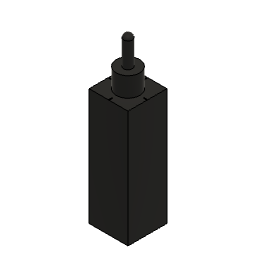
WW-PenMillReamerToolHolder (Autodesk Fusion 360 design; units mm, degrees)
Autodesk Fusion 360 part; units mm, degrees
sketch "Sketch1" plane through (0, 0, 0) normal (0, 1, 0) x (1, 0, 0) in component "Tool Holder - Whiteside"
  line L0 (0, 0) -> (25.4, 0)
  line L1 (25.4, 0) -> (25.4, -25.4)
  line L2 (25.4, -25.4) -> (0, -25.4)
  line L3 (0, -25.4) -> (0, 0)
  dimension "d1" = 25.4
  dimension "d2" = 25.4
  constraint horizontal L0
  constraint vertical L1
  constraint horizontal L2
  constraint vertical L3
  constraint coincident L0.start L3.end
  measures "d1" distance of L0.start L0.end
  measures "d2" distance of L0.start L2.end
extrude "Extrude1" add sketch "Sketch1" along normal blind 76.2 makes body 1 in component "Tool Holder - Whiteside"
sketch "Sketch2" plane through (0, 76.2, 0) normal (0, 1, 0) x (-1, 0, 0) in component "Tool Holder - Whiteside"
  line L0 (0, 25.4) -> (-25.4, 25.4)
  line L1 (-25.4, 25.4) -> (-25.4, 0)
  line L2 (-25.4, 0) -> (0, 0)
  line L3 (0, 0) -> (0, 25.4)
  line L4 (0, 25.4) -> (-12.7, 25.4)
  line L5 (-12.7, 25.4) -> (-12.7, 12.7)
  line L6 (-12.7, 12.7) -> (0, 12.7)
  line L7 (0, 12.7) -> (0, 25.4)
  circle A0 centre (-12.7, 12.7) radius 7.62
  dimension "d5" = 12.7
  dimension "d6" = 12.7
  dimension "d7" = 15.24
  constraint horizontal L4
  constraint vertical L5
  constraint horizontal L6
  constraint vertical L7
  constraint coincident L0.start L3.end
  constraint coincident L5.end L6.start
  measures "d5" distance of L0.start L4.end
  measures "d6" distance of L0.start L6.end
  measures "d7" diameter of A0
extrude "Extrude2" add sketch "Sketch2" along normal blind 12.7 contours L5 L6 A0 | L5 L6 A0 bodies 1 in component "Tool Holder - Whiteside"
sketch "Sketch3" plane through (0, 88.9, 0) normal (0, 1, 0) x (-1, 0, 0) in component "Tool Holder - Whiteside"
  circle A0 centre (-12.7, 12.7) radius 7.62
  circle A1 centre (-12.7, 12.7) radius 2.8575
  dimension "d10" = 5.715
  constraint concentric A0 A1
  measures "d10" diameter of A1
extrude "Extrude3" add sketch "Sketch3" along normal blind 19.05 contours A1 bodies 1 in component "Tool Holder - Whiteside"
chamfer "Chamfer1" distance 0.635 angle 45 1 edges at (15.3641, 107.95, 11.6667) on bodies 1 in component "Tool Holder - Whiteside"
chamfer "Chamfer2" distance 2.54 angle 45 3 edges at (25.4, 76.2, 12.7) (12.7, 76.2, 25.4) (0, 76.2, 12.7) on bodies 1 in component "Tool Holder - Whiteside"
fillet "Fillet1" radius 2.54 1 edges at (19.8043, 76.2, 15.4555) on bodies 1 in component "Tool Holder - Whiteside"
sketch "Sketch1 (2)" plane through (0, 0, 0) normal (0, 1, 0) x (1, 0, 0) in component "Milling Bit"
  circle A0 centre (-38.4906, 23.2969) radius 9.4361
  dimension "d17" = 18.8722
  measures "d17" diameter of A0
extrude "Extrude1'" add sketch "Sketch1 (2)" along normal blind 22.6568 separate body makes body 2 in component "Milling Bit"
sketch "Sketch2 (2)" plane through (0, 22.6568, 0) normal (0, 1, 0) x (-1, 0, 0) in component "Milling Bit"
  circle A0 centre (38.4906, -23.2969) radius 9.4361
  circle A1 centre (38.4906, -23.2969) radius 2.8702
  dimension "d20" = 5.7404
  constraint concentric A0 A1
  measures "d20" diameter of A1
extrude "Extrude2'" cut sketch "Sketch2 (2)" against normal blind 55.88 contours A1 bodies 2 in component "Milling Bit"
chamfer "Chamfer1'" distance 0.508 angle 45 1 edges at (-47.2881, 0, -19.8847) on bodies 2 in component "Milling Bit"
sketch "Sketch1 (3)" plane through (0, 111.5568, 0) normal (0, 1, 0) x (-1, 0, 0)
  circle A0 centre (-12.7067, 12.7059) radius 2.8702
  circle A1 centre (-12.7067, 12.7059) radius 9.4361
  line L0 (-12.7067, 12.7059) -> (-12.7067, 24.2231)
  line L1 (-12.7067, 24.2231) -> (-12.7067, 12.7059)
  line L2 (-12.7067, 1.8794) -> (-12.7067, 12.7059)
  line L3 (-12.7067, 12.7059) -> (-23.5469, 12.7059)
  line L4 (-12.7067, 12.7059) -> (-0.0671, 12.7059)
  line L5 (-12.7067, 12.7059) -> (-23.3575, 12.7059)
  line L6 (-23.3575, 12.7059) -> (-23.3575, 15.2459)
  line L7 (-23.3575, 15.2459) -> (-12.7067, 15.2459)
  line L8 (-12.7067, 15.2459) -> (-12.7067, 12.7059)
  line L9 (-12.7067, 12.7059) -> (-10.1667, 12.7059)
  line L10 (-10.1667, 12.7059) -> (-10.1667, 23.655)
  line L11 (-10.1667, 23.655) -> (-12.7067, 23.655)
  line L12 (-12.7067, 23.655) -> (-12.7067, 12.7059)
  line L13 (-12.7067, 12.7059) -> (-0.1302, 12.7059)
  line L14 (-0.1302, 12.7059) -> (-0.1302, 10.1659)
  line L15 (-0.1302, 10.1659) -> (-12.7067, 10.1659)
  line L16 (-12.7067, 10.1659) -> (-12.7067, 12.7059)
  line L17 (-12.7067, 12.7059) -> (-15.2467, 12.7059)
  line L18 (-15.2467, 12.7059) -> (-15.2467, 2.4475)
  line L19 (-15.2467, 2.4475) -> (-12.7067, 2.4475)
  line L20 (-12.7067, 2.4475) -> (-12.7067, 12.7059)
  dimension "d24" = 2.54
  dimension "d25" = 2.54
  dimension "d26" = 2.54
  dimension "d27" = 2.54
  constraint coincident A0.centre A1.centre
  constraint vertical L0
  constraint parallel L1 L2
  constraint perpendicular L0 L3
  constraint perpendicular L1 L4
  constraint horizontal L5
  constraint vertical L6
  constraint horizontal L7
  constraint vertical L8
  constraint horizontal L9
  constraint vertical L10
  constraint horizontal L11
  constraint vertical L12
  constraint horizontal L13
  constraint vertical L14
  constraint horizontal L15
  constraint vertical L16
  constraint horizontal L17
  constraint vertical L18
  constraint horizontal L19
  constraint vertical L20
  measures "d24" distance of A0.centre L7.end
  measures "d25" distance of A0.centre L9.end
  measures "d26" distance of A0.centre L15.end
  measures "d27" distance of A0.centre L17.end
extrude "Extrude3'" cut sketch "Sketch1 (3)" against normal blind 10.668 contours A0 A1 L4 L10 L13 | A0 A1 L2 L15 L20 | A0 A1 L0 L1 L7 L12 | A0 A1 L3 L5 L18 sketch seen with x (1, 0, 0) y (0, 1, 0) z (0, 0, 1) at (-51.1973, -88.9, -36.0029) bodies 2 in component "Milling Bit"
draft "Draft1" angle -10 neutral plane through (-35.6204, 22.6568, -23.2969) pull (0, 0, -1) 1 faces at (-31.3167, 22.6568, -22.3137) on bodies 2 in component "Milling Bit"
draft "Draft2" angle -10 neutral plane through (-38.4906, 22.6568, -32.733) pull (-1, 0, 0) 1 faces at (-37.5074, 22.6568, -30.4709) on bodies 2 in component "Milling Bit"
draft "Draft3" angle -10 neutral plane through (-41.3608, 22.6568, -23.2969) pull (0, 0, 1) 1 faces at (-45.6645, 22.6568, -24.2802) on bodies 2 in component "Milling Bit"
draft "Draft4" angle -10 neutral plane through (-38.4906, 22.6568, -20.4267) pull (1, 0, 0) 1 faces at (-39.4738, 22.6568, -16.123) on bodies 2 in component "Milling Bit"
chamfer "Chamfer2'" distance 10.16 distance2 6.858 1 edges at (-33.2784, 11.9888, -20.7569) measured on face at (-34.5703, 18.8022, -20.7569) on bodies 2 in component "Milling Bit"
chamfer "Chamfer3" distance 10.16 distance2 6.858 1 edges at (-35.9506, 11.9888, -28.5091) measured on face at (-35.9506, 18.8022, -29.801) on bodies 2 in component "Milling Bit"
chamfer "Chamfer4" distance 10.16 distance2 6.858 1 edges at (-43.7028, 11.9888, -25.8369) measured on face at (-42.4109, 15.3955, -25.8369) on bodies 2 in component "Milling Bit"
chamfer "Chamfer5" distance 10.16 distance2 6.858 1 edges at (-41.0306, 11.9888, -18.0847) measured on face at (-41.0306, 15.3955, -16.7929) on bodies 2 in component "Milling Bit"
sketch "Sketch1 (4)" plane through (0, 0, 0) normal (0, 1, 0) x (1, 0, 0) in component "Milling Bit 2"
  line L0 (-3.9, 2.8252) -> (21.5, 2.8252)
  line L1 (21.5, 2.8252) -> (21.5, -22.5748)
  line L2 (21.5, -22.5748) -> (-3.9, -22.5748)
  line L3 (-3.9, -22.5748) -> (-3.9, 2.8252)
  dimension "d46" = 25.4
  dimension "d47" = 25.4
  constraint horizontal L0
  constraint vertical L1
  constraint horizontal L2
  constraint vertical L3
  measures "d46" distance of L0.start L0.end
  measures "d47" distance of L0.start L2.end
extrude "Extrude1''" add sketch "Sketch1 (4)" along normal blind 25.4 separate body makes body 3 in component "Milling Bit 2"
sketch "Sketch2 (3)" plane through (0, 25.4, 0) normal (0, 1, 0) x (-1, 0, 0) in component "Milling Bit 2"
  line L0 (3.9, 22.5748) -> (-21.5, 22.5748)
  line L1 (-21.5, 22.5748) -> (-21.5, -2.8252)
  line L2 (-21.5, -2.8252) -> (3.9, -2.8252)
  line L3 (3.9, -2.8252) -> (3.9, 22.5748)
  line L4 (3.9, -2.8252) -> (-8.8, -2.8252)
  line L5 (-8.8, -2.8252) -> (-8.8, 9.8748)
  line L6 (-8.8, 9.8748) -> (3.9, 9.8748)
  line L7 (3.9, 9.8748) -> (3.9, -2.8252)
  line L8 (-8.8, 9.8748) -> (-6.26, 9.8748)
  line L9 (-6.26, 9.8748) -> (-6.26, 22.5748)
  line L10 (-6.26, 22.5748) -> (-8.8, 22.5748)
  line L11 (-8.8, 22.5748) -> (-8.8, 9.8748)
  line L12 (-8.8, 9.8748) -> (3.9, 9.8748)
  line L13 (3.9, 9.8748) -> (3.9, 7.3348)
  line L14 (3.9, 7.3348) -> (-8.8, 7.3348)
  line L15 (-8.8, 7.3348) -> (-8.8, 9.8748)
  line L16 (-8.8, 9.8748) -> (-11.34, 9.8748)
  line L17 (-11.34, 9.8748) -> (-11.34, -2.8252)
  line L18 (-11.34, -2.8252) -> (-8.8, -2.8252)
  line L19 (-8.8, -2.8252) -> (-8.8, 9.8748)
  line L20 (-8.8, 9.8748) -> (-21.5, 9.8748)
  line L21 (-21.5, 9.8748) -> (-21.5, 12.4148)
  line L22 (-21.5, 12.4148) -> (-8.8, 12.4148)
  line L23 (-8.8, 12.4148) -> (-8.8, 9.8748)
  dimension "d50" = 12.7
  dimension "d51" = 12.7
  dimension "d52" = 2.54
  dimension "d53" = 2.54
  dimension "d54" = 2.54
  dimension "d55" = 2.54
  constraint horizontal L4
  constraint vertical L5
  constraint horizontal L6
  constraint vertical L7
  constraint coincident L2.end L3.start
  constraint horizontal L8
  constraint vertical L9
  constraint horizontal L10
  constraint vertical L11
  constraint horizontal L12
  constraint vertical L13
  constraint horizontal L14
  constraint vertical L15
  constraint horizontal L16
  constraint vertical L17
  constraint horizontal L18
  constraint vertical L19
  constraint horizontal L20
  constraint vertical L21
  constraint horizontal L22
  constraint vertical L23
  measures "d50" distance of L2.end L4.end
  measures "d51" distance of L2.end L6.end
  measures "d52" distance of L5.end L8.end
  measures "d53" distance of L5.end L14.end
  measures "d54" distance of L5.end L16.end
  measures "d55" distance of L5.end L22.end
extrude "Extrude2''" cut sketch "Sketch2 (3)" against normal blind 10.414 contours L0 L3 L6 L9 L12 | L0 L1 L11 L22 | L2 L3 L4 L5 L7 L14 L19 | L1 L2 L17 L20 bodies 3 in component "Milling Bit 2"
sketch "Sketch3 (2)" plane through (8.8, 0, 0) normal (1, 0, 0) x (0, 0, -1) in component "Milling Bit 2"
  line L0 (-12.4148, 25.4) -> (-22.5748, 25.4)
  line L1 (-22.5748, 25.4) -> (-22.5748, 14.986)
  line L2 (-22.5748, 14.986) -> (-12.4148, 14.986)
  line L3 (-12.4148, 14.986) -> (-12.4148, 25.4)
  line L4 (-22.5748, 14.986) -> (-17.4948, 14.986)
  line L5 (-17.4948, 14.986) -> (-17.4948, 18.034)
  line L6 (-17.4948, 18.034) -> (-22.5748, 18.034)
  line L7 (-22.5748, 18.034) -> (-22.5748, 14.986)
  arc A0 (-22.5748, 14.986) -> (-12.4148, 25.4) centre (-28.9502, 31.369) ccw
  dimension "d58" = 5.08
  dimension "d59" = 3.048
  constraint horizontal L4
  constraint vertical L5
  constraint horizontal L6
  constraint vertical L7
  constraint coincident L1.end L2.start
  constraint coincident L5.end A0
  constraint coincident L0.start L3.end
  measures "d58" distance of L1.end L4.end
  measures "d59" distance of L1.end L6.end
extrude "Extrude3''" add sketch "Sketch3 (2)" along normal blind 12.7 contours L2 L3 L5 A0 | L2 L4 L5 A0 bodies 3 in component "Milling Bit 2"
sketch "Sketch4" plane through (0, 0, 9.8748) normal (0, 0, -1) x (-1, 0, 0) in component "Milling Bit 2"
  line L0 (-11.34, 25.4) -> (-21.5, 25.4)
  line L1 (-21.5, 25.4) -> (-21.5, 14.986)
  line L2 (-21.5, 14.986) -> (-11.34, 14.986)
  line L3 (-11.34, 14.986) -> (-11.34, 25.4)
  line L4 (-21.5, 14.986) -> (-16.42, 14.986)
  line L5 (-16.42, 14.986) -> (-16.42, 18.034)
  line L6 (-16.42, 18.034) -> (-21.5, 18.034)
  line L7 (-21.5, 18.034) -> (-21.5, 14.986)
  arc A0 (-21.5, 14.986) -> (-11.34, 25.4) centre (-27.8754, 31.369) ccw
  dimension "d62" = 5.08
  dimension "d63" = 3.048
  constraint horizontal L4
  constraint vertical L5
  constraint horizontal L6
  constraint vertical L7
  constraint coincident L1.end L2.start
  constraint coincident L5.end A0
  constraint coincident L0.start L3.end
  measures "d62" distance of L1.end L4.end
  measures "d63" distance of L1.end L6.end
extrude "Extrude4" add sketch "Sketch4" along normal blind 12.7 contours L2 L3 L5 A0 | L2 L4 L5 A0 bodies 3 in component "Milling Bit 2"
sketch "Sketch5" plane through (8.8, 0, 0) normal (-1, 0, 0) x (0, 0, 1) in component "Milling Bit 2"
  line L0 (7.3348, 25.4) -> (-2.8252, 25.4)
  line L1 (-2.8252, 25.4) -> (-2.8252, 14.986)
  line L2 (-2.8252, 14.986) -> (7.3348, 14.986)
  line L3 (7.3348, 14.986) -> (7.3348, 25.4)
  line L4 (-2.8252, 14.986) -> (2.2548, 14.986)
  line L5 (2.2548, 14.986) -> (2.2548, 18.034)
  line L6 (2.2548, 18.034) -> (-2.8252, 18.034)
  line L7 (-2.8252, 18.034) -> (-2.8252, 14.986)
  arc A0 (-2.8252, 14.986) -> (7.3348, 25.4) centre (-9.2006, 31.369) ccw
  dimension "d66" = 5.08
  dimension "d67" = 3.048
  constraint horizontal L4
  constraint vertical L5
  constraint horizontal L6
  constraint vertical L7
  constraint coincident L1.end L2.start
  constraint coincident L5.end A0
  constraint coincident L0.start L3.end
  measures "d66" distance of L1.end L4.end
  measures "d67" distance of L1.end L6.end
extrude "Extrude5" add sketch "Sketch5" along normal blind 12.7 contours L2 L3 L5 A0 | L2 L4 L5 A0 bodies 3 in component "Milling Bit 2"
sketch "Sketch6" plane through (0, 0, 9.8748) normal (0, 0, 1) x (1, 0, 0) in component "Milling Bit 2"
  line L0 (6.26, 25.4) -> (-3.9, 25.4)
  line L1 (-3.9, 25.4) -> (-3.9, 14.986)
  line L2 (-3.9, 14.986) -> (6.26, 14.986)
  line L3 (6.26, 14.986) -> (6.26, 25.4)
  line L4 (-3.9, 14.986) -> (1.18, 14.986)
  line L5 (1.18, 14.986) -> (1.18, 18.034)
  line L6 (1.18, 18.034) -> (-3.9, 18.034)
  line L7 (-3.9, 18.034) -> (-3.9, 14.986)
  arc A0 (-3.9, 14.986) -> (6.26, 25.4) centre (-10.2754, 31.369) ccw
  dimension "d70" = 5.08
  dimension "d71" = 3.048
  constraint horizontal L4
  constraint vertical L5
  constraint horizontal L6
  constraint vertical L7
  constraint coincident L1.end L2.start
  constraint coincident L5.end A0
  constraint coincident L0.start L3.end
  measures "d70" distance of L1.end L4.end
  measures "d71" distance of L1.end L6.end
extrude "Extrude6" add sketch "Sketch6" along normal blind 12.7 contours L2 L3 L5 A0 | L2 L4 L5 A0 bodies 3 in component "Milling Bit 2"
sketch "Sketch7" plane through (0, 0, 22.5748) normal (0, 0, 1) x (1, 0, 0) in component "Milling Bit 2"
  line L0 (-3.9, 14.986) -> (-3.9, 0)
  line L1 (-3.9, 0) -> (21.5, 0)
  line L2 (21.5, 0) -> (21.5, 14.986)
  line L3 (21.5, 14.986) -> (8.8, 14.986)
  line L4 (8.8, 14.986) -> (8.8, 25.4)
  line L5 (8.8, 25.4) -> (6.26, 25.4)
  arc A0 (-3.9, 14.986) -> (6.26, 25.4) centre (-10.2754, 31.369) ccw
  line L6 (8.8, 25.4) -> (3.9288, 24.5411)
  line L7 (8.8, 25.4) -> (13.7464, 25.4) construction
  dimension "d74" = 170
  constraint horizontal L7
  constraint coincident L4.end L5.start
  measures "d74" angle of L6 L7
extrude "Extrude7" cut sketch "Sketch7" against normal blind 12.7 contours L5 A0 L6 bodies 3 in component "Milling Bit 2"
sketch "Sketch8" plane through (21.5, 0, 0) normal (1, 0, 0) x (0, 0, -1) in component "Milling Bit 2"
  line L0 (-22.5748, 14.986) -> (-22.5748, 0)
  line L1 (-22.5748, 0) -> (2.8252, 0)
  line L2 (2.8252, 0) -> (2.8252, 14.986)
  line L3 (2.8252, 14.986) -> (-9.8748, 14.986)
  line L4 (-9.8748, 14.986) -> (-9.8748, 25.4)
  line L5 (-9.8748, 25.4) -> (-12.4148, 25.4)
  arc A0 (-22.5748, 14.986) -> (-12.4148, 25.4) centre (-28.9502, 31.369) ccw
  line L6 (-9.8748, 25.4) -> (-15.8886, 24.3396)
  line L7 (-9.8748, 25.4) -> (-3.7683, 25.4) construction
  dimension "d77" = 170
  constraint horizontal L7
  constraint coincident L4.end L5.start
  measures "d77" angle of L6 L7
extrude "Extrude8" cut sketch "Sketch8" against normal blind 12.7 contours L5 A0 L6 bodies 3 in component "Milling Bit 2"
sketch "Sketch9" plane through (0, 0, -2.8252) normal (0, 0, -1) x (-1, 0, 0) in component "Milling Bit 2"
  line L0 (-8.8, 14.986) -> (-8.8, 25.4)
  line L1 (-8.8, 25.4) -> (-11.34, 25.4)
  arc A0 (-21.5, 14.986) -> (-11.34, 25.4) centre (-27.8754, 31.369) ccw
  line L2 (-21.5, 14.986) -> (-21.5, 0)
  line L3 (-21.5, 0) -> (3.9, 0)
  line L4 (3.9, 0) -> (3.9, 14.986)
  line L5 (3.9, 14.986) -> (-8.8, 14.986)
  line L6 (-8.8, 25.4) -> (-15.2984, 24.2542)
  line L7 (-8.8, 25.4) -> (-2.2014, 25.4) construction
  dimension "d80" = 170
  constraint horizontal L7
  constraint coincident L0.end L1.start
  measures "d80" angle of L6 L7
extrude "Extrude9" cut sketch "Sketch9" against normal blind 12.7 contours L1 A0 L6 bodies 3 in component "Milling Bit 2"
sketch "Sketch10" plane through (-3.9, 0, 0) normal (-1, 0, 0) x (0, 0, 1) in component "Milling Bit 2"
  line L0 (22.5748, 14.986) -> (9.8748, 14.986)
  line L1 (9.8748, 14.986) -> (9.8748, 25.4)
  line L2 (9.8748, 25.4) -> (7.3348, 25.4)
  arc A0 (-2.8252, 14.986) -> (7.3348, 25.4) centre (-9.2006, 31.369) ccw
  line L3 (-2.8252, 14.986) -> (-2.8252, 0)
  line L4 (-2.8252, 0) -> (22.5748, 0)
  line L5 (22.5748, 0) -> (22.5748, 14.986)
  line L6 (9.8748, 25.4) -> (5.3598, 24.6039)
  line L7 (9.8748, 25.4) -> (14.4595, 25.4) construction
  dimension "d83" = 170
  constraint horizontal L7
  constraint coincident L1.end L2.start
  measures "d83" angle of L6 L7
extrude "Extrude10" cut sketch "Sketch10" against normal blind 12.7 contours L2 A0 L6 bodies 3 in component "Milling Bit 2"
sketch "Sketch11" plane through (0, 0, 0) normal (0, -1, 0) x (1, 0, 0) in component "Milling Bit 2"
  line L0 (21.5, 22.5748) -> (-3.9, 22.5748)
  line L1 (-3.9, 22.5748) -> (-3.9, -2.8252)
  line L2 (-3.9, -2.8252) -> (21.5, -2.8252)
  line L3 (21.5, -2.8252) -> (21.5, 22.5748)
  line L4 (-3.9, 22.5748) -> (8.8, 22.5748)
  line L5 (8.8, 22.5748) -> (8.8, 9.8748)
  line L6 (8.8, 9.8748) -> (-3.9, 9.8748)
  line L7 (-3.9, 9.8748) -> (-3.9, 22.5748)
  circle A0 centre (8.8, 9.8748) radius 9.525
  circle A1 centre (8.8, 9.8748) radius 2.8575
  dimension "d86" = 12.7
  dimension "d87" = 12.7
  dimension "d88" = 19.05
  dimension "d89" = 5.715
  constraint horizontal L4
  constraint vertical L5
  constraint horizontal L6
  constraint vertical L7
  constraint coincident L0.end L1.start
  constraint coincident L5.end L6.start
  constraint concentric A0 A1
  measures "d86" distance of L0.end L4.end
  measures "d87" distance of L0.end L6.end
  measures "d88" diameter of A0
  measures "d89" diameter of A1
extrude "Extrude11" cut sketch "Sketch11" against normal blind 40.64 contours L0 L1 L2 L3 L5 L6 A0 | L0 L1 L4 L5 L6 L7 A0 | L5 L6 A1 | L5 L6 A1 bodies 3 in component "Milling Bit 2"
chamfer "Chamfer3'" distance 2.54 distance2 2.54 1 edges at (12.7, 76.2, 0) measured on face at (12.4469, 76.2, 0.8561) on bodies 1 in component "Tool Holder - Whiteside"
delete_face "DeleteFace1" 4 faces at (12.7, 74.5067, 24.5533) (24.5533, 74.5067, 12.7) (12.7, 74.5067, 0.8467) (0.8467, 74.5067, 12.7) on bodies 1 in component "Tool Holder - Whiteside"
sketch "Sketch2 (4)" plane through (0, 76.2, 0) normal (0, 1, 0) x (-1, 0, 0)
  line L0 (0, 0) -> (0, 25.4)
  line L1 (0, 25.4) -> (-25.4, 25.4)
  line L2 (-25.4, 25.4) -> (-25.4, 0)
  line L3 (-25.4, 0) -> (0, 0)
  circle A0 centre (-12.7, 12.7) radius 10.16
  line L4 (-25.4, 25.4) -> (-12.7, 25.4)
  line L5 (-12.7, 25.4) -> (-12.7, 12.7)
  line L6 (-12.7, 12.7) -> (-25.4, 12.7)
  line L7 (-25.4, 12.7) -> (-25.4, 25.4)
  line L8 (-12.7, 12.7) -> (0, 12.7)
  line L9 (0, 12.7) -> (0, 0)
  line L10 (0, 0) -> (-12.7, 0)
  line L11 (-12.7, 0) -> (-12.7, 12.7)
  line L12 (-12.7, 0) -> (-12.9, 0)
  line L13 (-12.9, 0) -> (-12.9, 2.5569)
  line L14 (-12.9, 2.5569) -> (-12.7, 2.5569)
  line L15 (-12.7, 2.5569) -> (-12.7, 0)
  line L16 (-12.7, 0) -> (-12.5, 0)
  line L17 (-12.5, 0) -> (-12.5, 2.5663)
  line L18 (-12.5, 2.5663) -> (-12.7, 2.5663)
  line L19 (-12.7, 2.5663) -> (-12.7, 0)
  line L20 (0, 12.7) -> (-2.6109, 12.7)
  line L21 (-2.6109, 12.7) -> (-2.6109, 12.5)
  line L22 (-2.6109, 12.5) -> (0, 12.5)
  line L23 (0, 12.5) -> (0, 12.7)
  line L24 (0, 12.7) -> (-2.6109, 12.7)
  line L25 (-2.6109, 12.7) -> (-2.6109, 12.9)
  line L26 (-2.6109, 12.9) -> (0, 12.9)
  line L27 (0, 12.9) -> (0, 12.7)
  line L28 (-12.7, 25.4) -> (-12.5, 25.4)
  line L29 (-12.5, 25.4) -> (-12.5, 22.8464)
  line L30 (-12.5, 22.8464) -> (-12.7, 22.8464)
  line L31 (-12.7, 22.8464) -> (-12.7, 25.4)
  line L32 (-12.7, 25.4) -> (-12.9, 25.4)
  line L33 (-12.9, 25.4) -> (-12.9, 22.8464)
  line L34 (-12.9, 22.8464) -> (-12.7, 22.8464)
  line L35 (-12.7, 22.8464) -> (-12.7, 25.4)
  line L36 (-25.4, 12.7) -> (-22.8151, 12.7)
  line L37 (-22.8151, 12.7) -> (-22.8151, 12.5)
  line L38 (-22.8151, 12.5) -> (-25.4, 12.5)
  line L39 (-25.4, 12.5) -> (-25.4, 12.7)
  line L40 (-25.4, 12.7) -> (-22.8451, 12.7)
  line L41 (-22.8451, 12.7) -> (-22.8451, 12.9)
  line L42 (-22.8451, 12.9) -> (-25.4, 12.9)
  line L43 (-25.4, 12.9) -> (-25.4, 12.7)
  dimension "d94" = 12.7
  dimension "d95" = 0.2
  dimension "d96" = 0.2
  dimension "d97" = 0.2
  dimension "d98" = 0.2
  dimension "d99" = 0.2
  dimension "d100" = 0.2
  dimension "d101" = 0.2
  dimension "d102" = 0.2
  constraint horizontal L4
  constraint vertical L5
  constraint horizontal L6
  constraint vertical L7
  constraint coincident L1.end L2.start
  constraint horizontal L8
  constraint vertical L9
  constraint horizontal L10
  constraint vertical L11
  constraint coincident L0.start L3.end
  constraint coincident A0.centre L5.end
  constraint horizontal L12
  constraint vertical L13
  constraint horizontal L14
  constraint vertical L15
  constraint horizontal L16
  constraint vertical L17
  constraint horizontal L18
  constraint vertical L19
  constraint horizontal L20
  constraint vertical L21
  constraint horizontal L22
  constraint vertical L23
  constraint horizontal L24
  constraint vertical L25
  constraint horizontal L26
  constraint vertical L27
  constraint horizontal L28
  constraint vertical L29
  constraint horizontal L30
  constraint vertical L31
  constraint horizontal L32
  constraint vertical L33
  constraint horizontal L34
  constraint vertical L35
  constraint horizontal L36
  constraint vertical L37
  constraint horizontal L38
  constraint vertical L39
  constraint horizontal L40
  constraint vertical L41
  constraint horizontal L42
  constraint vertical L43
  measures "d94" distance of L1.end L6.end
  measures "d95" distance of L10.end L12.end
  measures "d96" distance of L10.end L16.end
  measures "d97" distance of L8.end L22.end
  measures "d98" distance of L8.end L26.end
  measures "d99" distance of L4.end L28.end
  measures "d100" distance of L4.end L32.end
  measures "d101" distance of L6.end L38.end
  measures "d102" distance of L6.end L42.end
extrude "Extrude4'" cut sketch "Sketch2 (4)" against normal blind 0.2 contours L0 A0 L8 L9 L20 L22 L23 L24 | L3 A0 L10 L11 L15 L16 L17 L19 | L0 A0 L8 L20 L24 L26 L27 | L3 A0 L11 L12 L13 L15 L19 | L1 A0 L5 L28 L29 L31 L35 | L2 A0 L6 L36 L38 L39 L40 | L1 A0 L4 L5 L31 L32 L33 L35 | L2 A0 L6 L7 L36 L40 L42 L43 bodies 1 in component "Tool Holder - Whiteside"
delete_face "DeleteFace2" 1 faces at (12.1112, 107.5267, 10.1205) on bodies 1 in component "Tool Holder - Whiteside"
fillet "Fillet2" radius 2.794 1 edges at (15.3641, 107.95, 13.7333) on bodies 1 in component "Tool Holder - Whiteside"
delete_face "DeleteFace3" 1 faces at (22.3673, 76.2459, 13.1825) on bodies 1 in component "Tool Holder - Whiteside"
component "Milling Bit" placed x (1, 0, 0) y (0, 1, 0) z (0, 0, 1) at (51.1973, 88.9, 36.0029)
component "Tool Holder - Whiteside" placed x (1, 0, 0) y (0, 1, 0) z (0, 0, 1) at (0, 0, 0)
component "Milling Bit 2" placed x (1, 0, 0) y (0, 1, 0) z (0, 0, 1) at (3.8853, 88.9, 2.8208)
